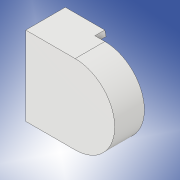
# Autodesk Inventor part: FA005
Saved by Autodesk Inventor 2017 SP1 (Build 210196100, 196)
## iProperties
Created: 2017-06-16
Part Number: FA005
Material: ABS Plastic
Document SubType Name: Modeling
Designer: Zach
Density: 1.06 g/cm^3
Appearance: CR White
Author: Zach
Autodesk Inventor part; units mm, degrees
ref_plane "YZ Plane" through (0, 0, 0) normal (1, 0, 0) x (0, 1, 0)
ref_plane "XZ Plane" through (0, 0, 0) normal (0, 1, 0) x (-1, 0, 0)
ref_plane "XY Plane" through (0, 0, 0) normal (0, 0, 1) x (1, 0, 0)
sketch "Sketch1" plane through (0, 0, 0) normal (0, 0, 1) x (1, 0, 0)
  line L0 (0, 0) -> (50, 0)
  line L1 (50, 0) -> (50, 80) construction
  line L2 (50, 80) -> (0, 80)
  line L3 (0, 80) -> (0, 0)
  circle A0 centre (50, 40) radius 40 construction
  arc A1 (50, 0) -> (50, 80) centre (50, 40) ccw
  dimension "d0" = 50
  dimension "d1" = 80
  dimension "d2" = 80
  constraints: 8 end point, 2 centre point, 2 parallel, 2 point on circle, 1 concentric, 1 horizontal, 1 midpoint, 1 perpendicular
  measures "d0" distance of L2.end L1.end
  measures "d1" distance of L1.end L0.end
  measures "d2" diameter of A0
extrude "Extrusion1" add sketch "Sketch1" along normal blind 40
sketch "Sketch2" plane through (0, 0, 0) normal (0, 0, -1) x (-1, 0, 0)
  line L0 (-50, 80) -> (0, 80) projected
  arc A0 (-50, 80) -> (-50, 0) centre (-50, 40) ccw projected
  line L1 (0, 0) -> (-50, 0) projected
  line L2 (0, 75) -> (-50, 75)
  arc A1 (-50, 75) -> (-50, 5) centre (-50, 40) ccw
  line L3 (-50, 5) -> (0, 5)
  line L4 (0, 75) -> (0, 5)
  line L5 (0, 80) -> (0, 0) projected
  dimension "d5" = 5
  constraints: 6 end point, 2 point on circle, 1 centre point, 1 collinear, 2 other
  measures "d5" distance between parallel lines of L0 L2
extrude "Extrusion2" cut sketch "Sketch2" against normal blind 35 contours L4 L3 A1 L2
sketch "Sketch3" plane through (0, 0, 40) normal (-1, 0, 0) x (0, 0, 1)
  line L0 (0, 80) -> (0, 0) projected
  line L1 (-40, 5) -> (-40, 75) projected
  line L2 (0, 80) -> (-40, 80)
  line L3 (-40, 80) -> (-40, 70)
  line L4 (-40, 70) -> (0, 70)
  line L5 (0, 70) -> (0, 80)
  line L6 (0, 80) -> (-10, 80)
  line L7 (-10, 80) -> (-10, 40)
  line L8 (-10, 40) -> (0, 40)
  line L9 (0, 40) -> (0, 80)
  line L10 (-40, 0) -> (0, 0) projected
  dimension "d8" = 10
  dimension "d9" = 10
  dimension "d10" = 40
  constraints: 16 end point, 4 parallel, 2 horizontal, 2 perpendicular, 1 point on line
  measures "d8" distance of L3.end L2.end
  measures "d9" distance of L8.end L7.end
  measures "d10" distance between parallel lines of L10 L8
extrude "Extrusion3" add sketch "Sketch3" against normal blind 5
sketch "Sketch4" plane through (0, 0, 0) normal (0, 0, -1) x (-1, 0, 0)
  arc A0 (-50, 80) -> (-50, 0) centre (-50, 40) ccw projected
  line L0 (-50, 80) -> (0, 80) projected
  arc A1 (-50, 80) -> (-50, 0) centre (-50, 40) ccw
  line L1 (-50, 0) -> (-50, 80)
  line L2 (-50, 40) -> (-40, 80)
  line L3 (-50, 80) -> (0, 80) projected
  line L4 (-40, 80) -> (-50, 80)
  line L5 (-50, 40) -> (-40, 0)
  line L6 (0, 0) -> (-50, 0) projected
  line L7 (-40, 0) -> (-50, 0)
  dimension "d15" = 10
  constraints: 10 end point, 2 collinear, 2 point on circle, 2 point on line, 1 centre point, 1 concentric, 1 vertical, 1 vertical alignment
  measures "d15" distance of L0.start L2.end
extrude "Extrusion4" cut sketch "Sketch4" against normal blind 10
body "Solid1"
